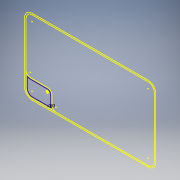
# Autodesk Inventor part: Hub Enclosure Front (new)
Saved by Autodesk Inventor 2018 (Build 220112000, 112)
## iProperties
Created: 2018-03-26
Part Number: Hub Enclosure Front (new)
Material: Generic
Document SubType Name: Modeling
Designer: brutu
Density: 1 g/cm^3
Appearance: Default
Author: brutu
Autodesk Inventor part; units mm, degrees
ref_plane "YZ Plane" through (0, 0, 0) normal (1, 0, 0) x (0, 1, 0)
ref_plane "XZ Plane" through (0, 0, 0) normal (0, 1, 0) x (-1, 0, 0)
ref_plane "XY Plane" through (0, 0, 0) normal (0, 0, 1) x (1, 0, 0)
sketch "Sketch1" plane through (0, 0, 0) normal (0, 0, 1) x (1, 0, 0)
  arc A0 (0, -0.381) -> (11, 10.619) centre (0, 10.619) ccw projected
  line L0 (11, 99.379) -> (11, 10.619) projected
  line L1 (0, -0.381) -> (-170.96, -0.381) projected
  arc A1 (11, 99.379) -> (0, 110.379) centre (0, 99.379) ccw projected
  line L2 (-170.96, 110.379) -> (0, 110.379) projected
  arc A2 (-170.96, 110.379) -> (-181.96, 99.379) centre (-170.96, 99.379) ccw projected
  line L3 (-181.96, 10.619) -> (-181.96, 99.379) projected
  arc A3 (-181.96, 10.619) -> (-170.96, -0.381) centre (-170.96, 10.619) ccw projected
  circle A4 centre (-22.38, 21.199) radius 1.5 projected
  circle A5 centre (-148.58, 21.199) radius 1.5 projected
  circle A6 centre (-148.58, 86.849) radius 1.5 projected
  circle A7 centre (-22.38, 86.849) radius 1.5 projected
  circle A8 centre (-22.38, 21.199) radius 1.905
  circle A9 centre (-22.38, 86.849) radius 1.905
  line L4 (-41.31, 1.719) -> (-129.65, 1.719)
  line L5 (-129.65, 108.279) -> (-41.31, 108.279)
  line L6 (8.9, 71.419) -> (8.9, 36.009)
  line L7 (-34.96, 23.309) -> (-34.96, 8.069)
  line L8 (-28.61, 29.659) -> (2.55, 29.659)
  arc A10 (-28.61, 29.659) -> (-34.96, 23.309) centre (-28.61, 23.309) ccw
  line L9 (2.55, 77.769) -> (-28.61, 77.769)
  line L10 (-34.96, 84.119) -> (-34.96, 101.929)
  arc A11 (-34.96, 84.119) -> (-28.61, 77.769) centre (-28.61, 84.119) ccw
  arc A12 (2.55, 29.659) -> (8.9, 36.009) centre (2.55, 36.009) ccw
  arc A13 (-41.31, 1.719) -> (-34.96, 8.069) centre (-41.31, 8.069) ccw
  arc A14 (-34.96, 101.929) -> (-41.31, 108.279) centre (-41.31, 101.929) ccw
  arc A15 (8.9, 71.419) -> (2.55, 77.769) centre (2.55, 71.419) ccw
  line L11 (-29.88, 25.199) -> (-29.88, 17.199) projected
  line L12 (-14.88, 25.199) -> (-29.88, 25.199) projected
  line L13 (-29.88, 82.849) -> (-14.88, 82.849) projected
  line L14 (-29.88, 90.849) -> (-29.88, 82.849) projected
  circle A16 centre (-148.58, 21.199) radius 1.905
  circle A17 centre (-148.58, 86.849) radius 1.905
  line L15 (-179.86, 71.419) -> (-179.86, 36.009)
  line L16 (-136, 23.309) -> (-136, 8.069)
  line L17 (-142.35, 29.659) -> (-173.51, 29.659)
  arc A18 (-136, 23.309) -> (-142.35, 29.659) centre (-142.35, 23.309) ccw
  line L18 (-173.51, 77.769) -> (-142.35, 77.769)
  line L19 (-136, 84.119) -> (-136, 101.929)
  arc A19 (-142.35, 77.769) -> (-136, 84.119) centre (-142.35, 84.119) ccw
  arc A20 (-179.86, 36.009) -> (-173.51, 29.659) centre (-173.51, 36.009) ccw
  arc A21 (-136, 8.069) -> (-129.65, 1.719) centre (-129.65, 8.069) ccw
  arc A22 (-129.65, 108.279) -> (-136, 101.929) centre (-129.65, 101.929) ccw
  arc A23 (-173.51, 77.769) -> (-179.86, 71.419) centre (-173.51, 71.419) ccw
  point P0 (0, 0)
  point P1 (-34.96, 1.719)
  point P2 (8.9, 29.659)
  point P3 (8.9, 77.769)
  point P4 (-34.96, 77.769)
  point P5 (-34.96, 108.279)
  dimension "d1" = 23.53
  dimension "d2" = 3.81
  dimension "d5" = 3.81
  dimension "d16" = 27.94
  dimension "d18" = 6.35
  dimension "d21" = 6.35
  dimension "d22" = 6.35
  dimension "d23" = 2.1
  dimension "d24" = 2.1
  dimension "d25" = 2.1
  dimension "d33" = 5.08
  dimension "d34" = 5.08
  dimension "d35" = 5.08
  dimension "d36" = 6.35
  dimension "d37" = 6.35
  constraints: 25 point on circle, 24 end point, 16 centre point, 12 tangent, 10 point on line, 2 coincident, 2 perpendicular, 1 equal radius, 1 horizontal, 1 vertical
  measures "d1" distance from line of L2 A7.centre
  measures "d2" diameter of A8
  measures "d5" diameter of A9
  measures "d16" distance between parallel lines of L4 L8
  measures "d18" radius of A10
  measures "d21" radius of A11
  measures "d22" radius of A12
  measures "d23" distance between parallel lines of L1 L4
  measures "d24" distance between parallel lines of L0 L6
  measures "d25" distance between parallel lines of L2 L5
  measures "d33" distance between parallel lines of L9 L13
  measures "d34" distance between parallel lines of L7 L11
  measures "d35" distance between parallel lines of L10 L14
  measures "d36" radius of A14
  measures "d37" radius of A15
extrude "Extrusion3" add sketch "Sketch1" along normal blind 2.1 contours L1 A3 L3 A2 L2 A1 L0 A0
sketch "Sketch4" plane through (0, 0, 2.1) normal (0, 0, 1) x (1, 0, 0)
  arc A0 (-28.61, 29.659) -> (-34.96, 23.309) centre (-28.61, 23.309) ccw projected
  line L0 (-34.96, 23.309) -> (-34.96, 8.069) projected
  arc A1 (-41.31, 1.719) -> (-34.96, 8.069) centre (-41.31, 8.069) ccw projected
  line L1 (-41.31, 1.719) -> (-129.65, 1.719) projected
  arc A2 (-136, 8.069) -> (-129.65, 1.719) centre (-129.65, 8.069) ccw projected
  line L2 (-136, 8.069) -> (-136, 23.309) projected
  arc A3 (-136, 23.309) -> (-142.35, 29.659) centre (-142.35, 23.309) ccw projected
  line L3 (-142.35, 29.659) -> (-173.51, 29.659) projected
  arc A4 (-179.86, 36.009) -> (-173.51, 29.659) centre (-173.51, 36.009) ccw projected
  line L4 (-179.86, 36.009) -> (-179.86, 71.419) projected
  arc A5 (-173.51, 77.769) -> (-179.86, 71.419) centre (-173.51, 71.419) ccw projected
  line L5 (-173.51, 77.769) -> (-142.35, 77.769) projected
  arc A6 (-142.35, 77.769) -> (-136, 84.119) centre (-142.35, 84.119) ccw projected
  line L6 (-136, 84.119) -> (-136, 101.929) projected
  arc A7 (-129.65, 108.279) -> (-136, 101.929) centre (-129.65, 101.929) ccw projected
  line L7 (-129.65, 108.279) -> (-41.31, 108.279) projected
  arc A8 (-34.96, 101.929) -> (-41.31, 108.279) centre (-41.31, 101.929) ccw projected
  line L8 (-34.96, 101.929) -> (-34.96, 84.119) projected
  arc A9 (-34.96, 84.119) -> (-28.61, 77.769) centre (-28.61, 84.119) ccw projected
  line L9 (-28.61, 77.769) -> (2.55, 77.769) projected
  arc A10 (8.9, 71.419) -> (2.55, 77.769) centre (2.55, 71.419) ccw projected
  line L10 (8.9, 71.419) -> (8.9, 36.009) projected
  arc A11 (2.55, 29.659) -> (8.9, 36.009) centre (2.55, 36.009) ccw projected
  line L11 (2.55, 29.659) -> (-28.61, 29.659) projected
  circle A12 centre (-148.58, 86.849) radius 1.905 projected
  circle A13 centre (-148.58, 21.199) radius 1.905 projected
  circle A14 centre (-22.38, 86.849) radius 1.905 projected
  circle A15 centre (-22.38, 21.199) radius 1.905 projected
  arc A16 (0, -0.381) -> (11, 10.619) centre (0, 10.619) ccw projected
  line L12 (11, 10.619) -> (11, 99.379) projected
  arc A17 (11, 99.379) -> (0, 110.379) centre (0, 99.379) ccw projected
  line L13 (0, 110.379) -> (-170.96, 110.379) projected
  arc A18 (-170.96, 110.379) -> (-181.96, 99.379) centre (-170.96, 99.379) ccw projected
  line L14 (-181.96, 99.379) -> (-181.96, 10.619) projected
  arc A19 (-181.96, 10.619) -> (-170.96, -0.381) centre (-170.96, 10.619) ccw projected
  line L15 (-170.96, -0.381) -> (0, -0.381) projected
  arc A20 (0, 1.719) -> (8.9, 10.619) centre (0, 10.619) ccw
  line L16 (8.9, 10.619) -> (8.9, 99.379)
  arc A21 (8.9, 99.379) -> (0, 108.279) centre (0, 99.379) ccw
  line L17 (0, 108.279) -> (-170.96, 108.279)
  arc A22 (-170.96, 108.279) -> (-179.86, 99.379) centre (-170.96, 99.379) ccw
  line L18 (-179.86, 99.379) -> (-179.86, 10.619)
  arc A23 (-179.86, 10.619) -> (-170.96, 1.719) centre (-170.96, 10.619) ccw
  line L19 (-170.96, 1.719) -> (0, 1.719)
  point P0 (0, 0)
  dimension "d40" = 2.1
  constraints: 8 end point, 8 point on circle, 4 centre point, 7 other
  measures "d40" distance between parallel lines of L15 L19
extrude "Extrusion4" add sketch "Sketch4" along normal blind 8.5 contours L15 A19 L14 A18 L13 A17 L12 A16
equation "\"d24\" = d23"
equation "\"d25\" = d23"
equation "\"d36\" = d22"
equation "\"d37\" = d22"
body "Solid2"
